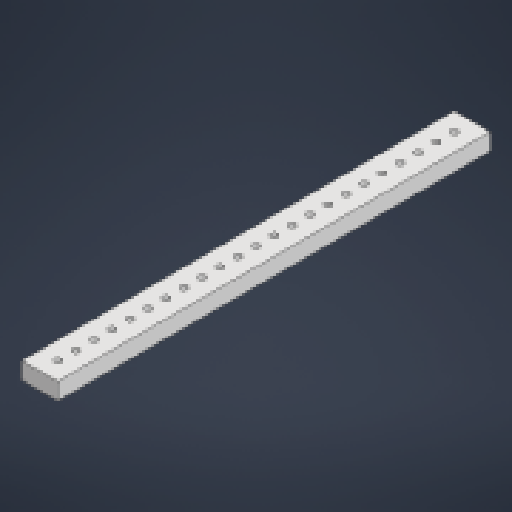
# Autodesk Inventor part: linkage
Saved by Autodesk Inventor 2023 (Build 270158000, 158)
## iProperties
Created: 2023-01-24
Part Number: linkage
Material: Generic
Document SubType Name: Modeling
Designer: Blank Slate
Density: 1 g/cm^3
Appearance: Default
Author: Blank Slate
Autodesk Inventor part; units mm, degrees
ref_plane "YZ Plane" through (0, 0, 0) normal (1, 0, 0) x (0, 1, 0)
ref_plane "XZ Plane" through (0, 0, 0) normal (0, 1, 0) x (-1, 0, 0)
ref_plane "XY Plane" through (0, 0, 0) normal (0, 0, 1) x (1, 0, 0)
sketch "Sketch1" plane through (0, 0, 0) normal (0, 1, 0) x (-1, 0, 0)
  line L0 (-344.259, 333.63) -> (-369.659, 333.63)
  line L1 (-369.659, 333.63) -> (-369.659, 28.83)
  line L2 (-369.659, 28.83) -> (-344.259, 28.83)
  line L3 (-344.259, 28.83) -> (-344.259, 333.63)
  point P0 (0, 0)
  dimension "d0" = 25.4
  dimension "d1" = 304.8
  constraints: 8 end point, 2 parallel, 1 horizontal, 1 perpendicular
  measures "d0" distance of L2.end L1.end
  measures "d1" distance of L1.end L0.end
extrude "Extrusion1" add sketch "Sketch1" along normal blind 11.938
sketch "Sketch2" plane through (0, 11.938, 0) normal (0, 1, 0) x (1, 0, 0)
  line L0 (369.659, -28.83) -> (344.259, -28.83) projected
  line L1 (356.959, -28.83) -> (356.959, -333.63) construction
  circle A0 centre (356.959, -41.53) radius 2.3813
  circle A1 centre (356.959, -54.23) radius 2.3813
  circle A2 centre (356.959, -66.93) radius 2.3813
  circle A3 centre (356.959, -79.63) radius 2.3813
  circle A4 centre (356.959, -92.33) radius 2.3813
  circle A5 centre (356.959, -105.03) radius 2.3813
  circle A6 centre (356.959, -117.73) radius 2.3813
  circle A7 centre (356.959, -130.43) radius 2.3813
  circle A8 centre (356.959, -143.13) radius 2.3813
  circle A9 centre (356.959, -155.83) radius 2.3813
  circle A10 centre (356.959, -168.53) radius 2.3813
  circle A11 centre (356.959, -181.23) radius 2.3813
  circle A12 centre (356.959, -193.93) radius 2.3813
  circle A13 centre (356.959, -206.63) radius 2.3813
  circle A14 centre (356.959, -219.33) radius 2.3813
  circle A15 centre (356.959, -232.03) radius 2.3813
  circle A16 centre (356.959, -244.73) radius 2.3813
  circle A17 centre (356.959, -257.43) radius 2.3813
  circle A18 centre (356.959, -270.13) radius 2.3813
  circle A19 centre (356.959, -282.83) radius 2.3813
  circle A20 centre (356.959, -295.53) radius 2.3813
  circle A21 centre (356.959, -308.23) radius 2.3813
  circle A22 centre (356.959, -320.93) radius 2.3813
  point P0 (0, 0)
  dimension "d20" = 4.7625
  dimension "d21" = 12.7
  dimension "d24" = 12.7
  constraints: 23 centre point, 2 end point, 2 midpoint, 2 vertical, 1 point on line, 44 other
  measures "d20" diameter of A0
  measures "d21" distance of point (356.959, -28.83) A0.centre
  measures "d24" distance of A0.centre A1.centre
hole "Hole1" at (356.959, 11.938, 41.53) at (356.959, 11.938, 54.23) at (356.959, 11.938, 66.93) at (356.959, 11.938, 79.63) at (356.959, 11.938, 92.33) at (356.959, 11.938, 105.03) at (356.959, 11.938, 117.73) at (356.959, 11.938, 130.43) at (356.959, 11.938, 143.13) at (356.959, 11.938, 155.83) at (356.959, 11.938, 168.53) at (356.959, 11.938, 181.23) at (356.959, 11.938, 193.93) at (356.959, 11.938, 206.63) at (356.959, 11.938, 219.33) at (356.959, 11.938, 232.03) at (356.959, 11.938, 244.73) at (356.959, 11.938, 257.43) at (356.959, 11.938, 270.13) at (356.959, 11.938, 282.83) at (356.959, 11.938, 295.53) at (356.959, 11.938, 308.23) at (356.959, 11.938, 320.93) direction (0, -1, 0) diameter 4.7625 end through all
body "Solid1"
